Autodesk Fusion 360 part; units mm, degrees
(part 3 of 3)
  arc A621 (50.492, 81.2182) -> (50.5682, 81.142) centre (50.5682, 81.2182) ccw
  line L959 (43.8912, 86.448) -> (44.7548, 86.448)
  line L960 (109.4275, 91.606) -> (110.2911, 91.606)
  line L961 (73.826, 73.9902) -> (73.826, 74.8538)
  arc A622 (123.8293, 93.7142) -> (123.9055, 93.638) centre (123.9055, 93.7142) ccw
  line L962 (110.3673, 91.6822) -> (110.3673, 92.5458)
  arc A623 (123.9055, 96.354) -> (123.8293, 96.2778) centre (123.9055, 96.2778) ccw
  arc A624 (53.0682, 87.858) -> (52.992, 87.7818) centre (53.0682, 87.7818) ccw
  line L963 (91.401, 91.6178) -> (91.401, 90.7542)
  arc A625 (122.8133, 96.2778) -> (122.7371, 96.354) centre (122.7371, 96.2778) ccw
  arc A626 (121.8735, 94.654) -> (121.7973, 94.5778) centre (121.8735, 94.5778) ccw
  arc A627 (122.7371, 95.338) -> (122.8133, 95.4142) centre (122.7371, 95.4142) ccw
  line L964 (124.8453, 95.4142) -> (124.8453, 96.2778)
  arc A628 (52.992, 86.9182) -> (53.0682, 86.842) centre (53.0682, 86.9182) ccw
  arc A629 (122.7371, 93.638) -> (122.8133, 93.7142) centre (122.7371, 93.7142) ccw
  line L965 (123.9055, 93.638) -> (124.7691, 93.638)
  arc A630 (92.417, 91.6178) -> (92.3408, 91.694) centre (92.3408, 91.6178) ccw
  arc A631 (52.992, 85.2182) -> (53.0682, 85.142) centre (53.0682, 85.2182) ccw
  line L966 (121.8735, 93.638) -> (122.7371, 93.638)
  arc A632 (109.4275, 92.622) -> (109.3513, 92.5458) centre (109.4275, 92.5458) ccw
  line L967 (51.4318, 82.158) -> (50.5682, 82.158)
  arc A633 (91.401, 90.7542) -> (91.4772, 90.678) centre (91.4772, 90.7542) ccw
  line L968 (121.7973, 96.2778) -> (121.7973, 95.4142)
  arc A634 (89.701, 90.7542) -> (89.7772, 90.678) centre (89.7772, 90.7542) ccw
  line L969 (52.992, 87.7818) -> (52.992, 86.9182)
  arc A635 (44.7548, 86.448) -> (44.831, 86.5242) centre (44.7548, 86.5242) ccw
  line L970 (53.0682, 85.142) -> (53.9318, 85.142)
  line L971 (75.4498, 74.93) -> (74.5862, 74.93)
  line L972 (44.7548, 87.464) -> (43.8912, 87.464)
  arc A636 (43.8912, 87.464) -> (43.815, 87.3878) centre (43.8912, 87.3878) ccw
  arc A637 (75.526, 74.8538) -> (75.4498, 74.93) centre (75.4498, 74.8538) ccw
  line L973 (121.8735, 95.338) -> (122.7371, 95.338)
  arc A638 (109.4275, 94.322) -> (109.3513, 94.2458) centre (109.4275, 94.2458) ccw
  line L974 (109.3513, 94.2458) -> (109.3513, 93.3822)
  arc A639 (50.5682, 83.858) -> (50.492, 83.7818) centre (50.5682, 83.7818) ccw
  arc A640 (91.4772, 91.694) -> (91.401, 91.6178) centre (91.4772, 91.6178) ccw
  arc A641 (72.81, 73.9902) -> (72.8862, 73.914) centre (72.8862, 73.9902) ccw
  line L975 (91.4772, 90.678) -> (92.3408, 90.678)
  line L976 (109.3513, 92.5458) -> (109.3513, 91.6822)
  line L977 (124.8453, 93.7142) -> (124.8453, 94.5778)
  arc A642 (81.2292, 72.859) -> (81.153, 72.7828) centre (81.2292, 72.7828) ccw
  arc A643 (43.8912, 85.764) -> (43.815, 85.6878) centre (43.8912, 85.6878) ccw
  arc A644 (109.3513, 91.6822) -> (109.4275, 91.606) centre (109.4275, 91.6822) ccw
  line L978 (43.8912, 84.748) -> (44.7548, 84.748)
  arc A645 (110.2911, 93.306) -> (110.3673, 93.3822) centre (110.2911, 93.3822) ccw
  arc A646 (123.9055, 94.654) -> (123.8293, 94.5778) centre (123.9055, 94.5778) ccw
  line L979 (123.8293, 96.2778) -> (123.8293, 95.4142)
  line L980 (53.9318, 86.158) -> (53.0682, 86.158)
  line L981 (72.81, 74.8538) -> (72.81, 73.9902)
  arc A647 (124.8453, 96.2778) -> (124.7691, 96.354) centre (124.7691, 96.2778) ccw
  arc A648 (44.7548, 84.748) -> (44.831, 84.8242) centre (44.7548, 84.8242) ccw
  line L982 (89.7772, 90.678) -> (90.6408, 90.678)
  arc A649 (98.314, 111.517) -> (98.209, 111.412) centre (98.314, 111.412) ccw
  line L983 (120.777, 70.6492) -> (120.777, 71.5128)
  line L984 (120.7051, 94.654) -> (119.8415, 94.654)
  arc A650 (95.209, 109.822) -> (95.314, 109.717) centre (95.314, 109.822) ccw
  line L985 (120.7813, 93.7142) -> (120.7813, 94.5778)
  arc A651 (109.3513, 93.3822) -> (109.4275, 93.306) centre (109.4275, 93.3822) ccw
  line L986 (123.9055, 95.338) -> (124.7691, 95.338)
  line L987 (120.7008, 71.589) -> (119.8372, 71.589)
  arc A652 (119.8415, 94.654) -> (119.7653, 94.5778) centre (119.8415, 94.5778) ccw
  arc A653 (95.314, 111.517) -> (95.209, 111.412) centre (95.314, 111.412) ccw
  line L988 (119.761, 69.8128) -> (119.761, 68.9492)
  arc A654 (116.6009, 119.19) -> (116.7059, 119.085) centre (116.7059, 119.19) ccw
  line L989 (122.8133, 95.4142) -> (122.8133, 96.2778)
  line L990 (92.3408, 91.694) -> (91.4772, 91.694)
  arc A655 (120.7813, 94.5778) -> (120.7051, 94.654) centre (120.7051, 94.5778) ccw
  arc A656 (121.7973, 95.4142) -> (121.8735, 95.338) centre (121.8735, 95.4142) ccw
  arc A657 (119.8372, 69.889) -> (119.761, 69.8128) centre (119.8372, 69.8128) ccw
  arc A658 (120.777, 69.8128) -> (120.7008, 69.889) centre (120.7008, 69.8128) ccw
  arc A659 (119.7653, 93.7142) -> (119.8415, 93.638) centre (119.8415, 93.7142) ccw
  line L991 (90.717, 90.7542) -> (90.717, 91.6178)
  line L992 (89.701, 91.6178) -> (89.701, 90.7542)
  line L993 (122.7371, 96.354) -> (121.8735, 96.354)
  arc A660 (121.7973, 93.7142) -> (121.8735, 93.638) centre (121.8735, 93.7142) ccw
  arc A661 (124.7691, 93.638) -> (124.8453, 93.7142) centre (124.7691, 93.7142) ccw
  line L994 (98.209, 111.412) -> (98.209, 109.822)
  arc A662 (89.7772, 91.694) -> (89.701, 91.6178) centre (89.7772, 91.6178) ccw
  line L995 (124.7691, 96.354) -> (123.9055, 96.354)
  line L996 (109.4275, 93.306) -> (110.2911, 93.306)
  line L997 (119.8415, 93.638) -> (120.7051, 93.638)
  arc A663 (118.4009, 120.38) -> (118.2959, 120.485) centre (118.2959, 120.38) ccw
  line L998 (118.2959, 123.485) -> (116.7059, 123.485)
  arc A664 (116.7059, 120.485) -> (116.6009, 120.38) centre (116.7059, 120.38) ccw
  arc A665 (119.761, 68.9492) -> (119.8372, 68.873) centre (119.8372, 68.9492) ccw
  line L999 (116.7059, 122.085) -> (118.2959, 122.085)
  arc A666 (124.7691, 95.338) -> (124.8453, 95.4142) centre (124.7691, 95.4142) ccw
  arc A667 (92.3408, 90.678) -> (92.417, 90.7542) centre (92.3408, 90.7542) ccw
  line L1000 (121.7973, 94.5778) -> (121.7973, 93.7142)
  arc A668 (120.7008, 70.573) -> (120.777, 70.6492) centre (120.7008, 70.6492) ccw
  arc A669 (120.7051, 95.338) -> (120.7813, 95.4142) centre (120.7051, 95.4142) ccw
  line L1001 (122.7371, 94.654) -> (121.8735, 94.654)
  line L1002 (119.761, 71.5128) -> (119.761, 70.6492)
  arc A670 (121.8735, 96.354) -> (121.7973, 96.2778) centre (121.8735, 96.2778) ccw
  line L1003 (124.7691, 94.654) -> (123.9055, 94.654)
  arc A671 (120.777, 71.5128) -> (120.7008, 71.589) centre (120.7008, 71.5128) ccw
  line L1004 (96.504, 111.517) -> (95.314, 111.517)
  line L1005 (116.7059, 119.085) -> (118.2959, 119.085)
  arc A672 (116.7059, 123.485) -> (116.6009, 123.38) centre (116.7059, 123.38) ccw
  arc A673 (120.7051, 93.638) -> (120.7813, 93.7142) centre (120.7051, 93.7142) ccw
  line L1006 (119.8372, 70.573) -> (120.7008, 70.573)
  line L1007 (119.7653, 96.2778) -> (119.7653, 95.4142)
  line L1008 (120.777, 68.9492) -> (120.777, 69.8128)
  arc A674 (98.209, 109.822) -> (98.314, 109.717) centre (98.314, 109.822) ccw
  arc A675 (123.8293, 95.4142) -> (123.9055, 95.338) centre (123.9055, 95.4142) ccw
  arc A676 (122.8133, 94.5778) -> (122.7371, 94.654) centre (122.7371, 94.5778) ccw
  arc A677 (118.2959, 119.085) -> (118.4009, 119.19) centre (118.2959, 119.19) ccw
  arc A678 (119.8415, 96.354) -> (119.7653, 96.2778) centre (119.8415, 96.2778) ccw
  line L1009 (118.4009, 119.19) -> (118.4009, 120.38)
  line L1010 (116.6009, 123.38) -> (116.6009, 122.19)
  arc A679 (110.3673, 92.5458) -> (110.2911, 92.622) centre (110.2911, 92.5458) ccw
  line L1011 (99.609, 109.822) -> (99.609, 111.412)
  line L1012 (120.7813, 95.4142) -> (120.7813, 96.2778)
  line L1013 (122.8133, 93.7142) -> (122.8133, 94.5778)
  arc A680 (99.504, 109.717) -> (99.609, 109.822) centre (99.504, 109.822) ccw
  line L1014 (110.3673, 93.3822) -> (110.3673, 94.2458)
  line L1015 (124.7648, 69.889) -> (123.9012, 69.889)
  line L1016 (110.5408, 69.508) -> (109.6772, 69.508)
  arc A681 (116.6009, 122.19) -> (116.7059, 122.085) centre (116.7059, 122.19) ccw
  line L1017 (123.825, 71.5128) -> (123.825, 70.6492)
  line L1018 (120.7051, 96.354) -> (119.8415, 96.354)
  line L1019 (116.6009, 120.38) -> (116.6009, 119.19)
  line L1020 (79.375, 116.7502) -> (79.375, 117.6138)
  arc A682 (79.375, 117.6138) -> (79.2988, 117.69) centre (79.2988, 117.6138) ccw
  arc A683 (78.4352, 117.69) -> (78.359, 117.6138) centre (78.4352, 117.6138) ccw
  line L1021 (120.7008, 69.889) -> (119.8372, 69.889)
  line L1022 (109.6772, 68.492) -> (110.5408, 68.492)
  arc A684 (123.825, 70.6492) -> (123.9012, 70.573) centre (123.9012, 70.6492) ccw
  line L1023 (95.209, 111.412) -> (95.209, 109.822)
  arc A685 (120.7008, 68.873) -> (120.777, 68.9492) centre (120.7008, 68.9492) ccw
  arc A686 (96.609, 111.412) -> (96.504, 111.517) centre (96.504, 111.412) ccw
  line L1024 (118.2959, 120.485) -> (116.7059, 120.485)
  arc A687 (78.359, 116.7502) -> (78.4352, 116.674) centre (78.4352, 116.7502) ccw
  arc A688 (124.841, 69.8128) -> (124.7648, 69.889) centre (124.7648, 69.8128) ccw
  line L1025 (121.8692, 70.573) -> (122.7328, 70.573)
  line L1026 (96.609, 109.822) -> (96.609, 111.412)
  arc A689 (110.2911, 91.606) -> (110.3673, 91.6822) centre (110.2911, 91.6822) ccw
  arc A690 (121.8692, 69.889) -> (121.793, 69.8128) centre (121.8692, 69.8128) ccw
  line L1027 (124.841, 70.6492) -> (124.841, 71.5128)
  arc A691 (121.8692, 71.589) -> (121.793, 71.5128) centre (121.8692, 71.5128) ccw
  arc A692 (109.6772, 69.508) -> (109.601, 69.4318) centre (109.6772, 69.4318) ccw
  arc A693 (124.7648, 70.573) -> (124.841, 70.6492) centre (124.7648, 70.6492) ccw
  arc A694 (110.5408, 68.492) -> (110.617, 68.5682) centre (110.5408, 68.5682) ccw
  arc A695 (96.504, 109.717) -> (96.609, 109.822) centre (96.504, 109.822) ccw
  line L1028 (124.7648, 71.589) -> (123.9012, 71.589)
  line L1029 (122.7328, 69.889) -> (121.8692, 69.889)
  line L1030 (119.8415, 95.338) -> (120.7051, 95.338)
  line L1031 (110.617, 68.5682) -> (110.617, 69.4318)
  line L1032 (118.4009, 122.19) -> (118.4009, 123.38)
  line L1033 (121.793, 71.5128) -> (121.793, 70.6492)
  line L1034 (99.504, 111.517) -> (98.314, 111.517)
  arc A696 (119.761, 70.6492) -> (119.8372, 70.573) centre (119.8372, 70.6492) ccw
  arc A697 (122.7328, 68.873) -> (122.809, 68.9492) centre (122.7328, 68.9492) ccw
  arc A698 (99.609, 111.412) -> (99.504, 111.517) centre (99.504, 111.412) ccw
  line L1035 (119.7653, 94.5778) -> (119.7653, 93.7142)
  arc A699 (119.7653, 95.4142) -> (119.8415, 95.338) centre (119.8415, 95.4142) ccw
  arc A700 (123.825, 68.9492) -> (123.9012, 68.873) centre (123.9012, 68.9492) ccw
  line L1036 (78.359, 115.9138) -> (78.359, 115.0502)
  line L1037 (109.6772, 70.192) -> (110.5408, 70.192)
  arc A701 (119.8372, 71.589) -> (119.761, 71.5128) centre (119.8372, 71.5128) ccw
  arc A702 (118.2959, 122.085) -> (118.4009, 122.19) centre (118.2959, 122.19) ccw
  arc A703 (123.9012, 71.589) -> (123.825, 71.5128) centre (123.9012, 71.5128) ccw
  arc A704 (109.601, 68.5682) -> (109.6772, 68.492) centre (109.6772, 68.5682) ccw
  line L1038 (98.314, 109.717) -> (99.504, 109.717)
  arc A705 (121.793, 68.9492) -> (121.8692, 68.873) centre (121.8692, 68.9492) ccw
  arc A706 (109.6772, 71.208) -> (109.601, 71.1318) centre (109.6772, 71.1318) ccw
  line L1039 (95.314, 109.717) -> (96.504, 109.717)
  line L1040 (78.4352, 114.974) -> (79.2988, 114.974)
  arc A707 (118.4009, 123.38) -> (118.2959, 123.485) centre (118.2959, 123.38) ccw
  arc A708 (78.4352, 115.99) -> (78.359, 115.9138) centre (78.4352, 115.9138) ccw
  arc A709 (78.359, 115.0502) -> (78.4352, 114.974) centre (78.4352, 115.0502) ccw
  line L1041 (123.9012, 68.873) -> (124.7648, 68.873)
  line L1042 (122.809, 68.9492) -> (122.809, 69.8128)
  line L1043 (122.7328, 71.589) -> (121.8692, 71.589)
  line L1044 (109.601, 71.1318) -> (109.601, 70.2682)
  arc A710 (124.841, 71.5128) -> (124.7648, 71.589) centre (124.7648, 71.5128) ccw
  line L1045 (119.8372, 68.873) -> (120.7008, 68.873)
  arc A711 (120.7813, 96.2778) -> (120.7051, 96.354) centre (120.7051, 96.2778) ccw
  line L1046 (121.793, 69.8128) -> (121.793, 68.9492)
  line L1047 (79.2988, 117.69) -> (78.4352, 117.69)
  line L1048 (66.928, 77.135) -> (66.028, 77.135)
  line L1049 (46.909, 73.405) -> (46.309, 73.405)
  line L1050 (47.859, 71.005) -> (47.259, 71.005)
  line L1051 (63.628, 78.085) -> (63.628, 77.485)
  arc A712 (110.5408, 70.192) -> (110.617, 70.2682) centre (110.5408, 70.2682) ccw
  line L1052 (45.959, 71.005) -> (45.359, 71.005)
  line L1053 (83.914, 118.45) -> (85.504, 118.45)
  line L1054 (46.309, 72.505) -> (46.909, 72.505)
  line L1055 (45.359, 70.105) -> (45.959, 70.105)
  arc A713 (85.504, 121.45) -> (85.609, 121.555) centre (85.504, 121.555) ccw
  line L1056 (46.25, 81.25) -> (45.65, 81.25)
  line L1057 (109.601, 69.4318) -> (109.601, 68.5682)
  arc A714 (121.793, 70.6492) -> (121.8692, 70.573) centre (121.8692, 70.6492) ccw
  arc A715 (110.617, 71.1318) -> (110.5408, 71.208) centre (110.5408, 71.1318) ccw
  arc A716 (122.809, 71.5128) -> (122.7328, 71.589) centre (122.7328, 71.5128) ccw
  line L1058 (78.4352, 116.674) -> (79.2988, 116.674)
  line L1059 (66.028, 76.185) -> (66.028, 75.585)
  line L1060 (110.617, 70.2682) -> (110.617, 71.1318)
  line L1061 (66.028, 76.535) -> (66.928, 76.535)
  arc A717 (66.628, 77.485) -> (66.628, 78.085) centre (66.628, 77.785) ccw
  line L1062 (66.028, 77.135) -> (66.028, 76.535)
  line L1063 (122.809, 70.6492) -> (122.809, 71.5128)
  line L1064 (63.628, 77.485) -> (64.528, 77.485)
  line L1065 (46.909, 72.505) -> (46.909, 73.405)
  arc A718 (109.601, 70.2682) -> (109.6772, 70.192) centre (109.6772, 70.2682) ccw
  line L1066 (123.9012, 70.573) -> (124.7648, 70.573)
  line L1067 (47.259, 73.405) -> (47.259, 72.505)
  line L1068 (43.75, 80.35) -> (44.35, 80.35)
  line L1069 (124.841, 68.9492) -> (124.841, 69.8128)
  line L1070 (123.825, 69.8128) -> (123.825, 68.9492)
  line L1071 (121.8692, 68.873) -> (122.7328, 68.873)
  arc A719 (122.809, 69.8128) -> (122.7328, 69.889) centre (122.7328, 69.8128) ccw
  line L1072 (63.628, 75.585) -> (64.528, 75.585)
  arc A720 (124.7648, 68.873) -> (124.841, 68.9492) centre (124.7648, 68.9492) ccw
  arc A721 (83.809, 118.555) -> (83.914, 118.45) centre (83.914, 118.555) ccw
  line L1073 (45.359, 72.805) -> (45.359, 73.105)
  line L1074 (64.528, 78.085) -> (63.628, 78.085)
  arc A722 (123.9012, 69.889) -> (123.825, 69.8128) centre (123.9012, 69.8128) ccw
  arc A723 (110.617, 69.4318) -> (110.5408, 69.508) centre (110.5408, 69.4318) ccw
  line L1075 (47.859, 73.405) -> (47.259, 73.405)
  line L1076 (110.5408, 71.208) -> (109.6772, 71.208)
  arc A724 (83.809, 121.555) -> (83.914, 121.45) centre (83.914, 121.555) ccw
  arc A725 (122.7328, 70.573) -> (122.809, 70.6492) centre (122.7328, 70.6492) ccw
  arc A726 (85.609, 119.745) -> (85.504, 119.85) centre (85.504, 119.745) ccw
  line L1077 (79.2988, 115.99) -> (78.4352, 115.99)
  line L1078 (78.359, 117.6138) -> (78.359, 116.7502)
  line L1079 (45.959, 72.805) -> (45.959, 73.105)
  line L1080 (64.528, 75.585) -> (64.528, 76.185)
  line L1081 (85.609, 121.555) -> (85.609, 122.745)
  line L1082 (47.859, 70.105) -> (47.859, 71.005)
  line L1083 (66.328, 78.085) -> (66.628, 78.085)
  line L1084 (66.328, 77.485) -> (66.628, 77.485)
  line L1085 (79.375, 115.0502) -> (79.375, 115.9138)
  line L1086 (83.809, 122.745) -> (83.809, 121.555)
  line L1087 (66.028, 75.585) -> (66.928, 75.585)
  line L1088 (64.528, 77.485) -> (64.528, 78.085)
  line L1089 (47.259, 70.105) -> (47.859, 70.105)
  line L1090 (66.928, 76.535) -> (66.928, 77.135)
  arc A727 (79.2988, 116.674) -> (79.375, 116.7502) centre (79.2988, 116.7502) ccw
  arc A728 (45.959, 73.105) -> (45.359, 73.105) centre (45.659, 73.105) ccw
  line L1091 (85.504, 119.85) -> (83.914, 119.85)
  line L1092 (64.528, 76.185) -> (63.628, 76.185)
  line L1093 (46.309, 73.405) -> (46.309, 72.505)
  line L1094 (63.628, 76.185) -> (63.628, 75.585)
  line L1095 (119.4533, 90.99) -> (119.8533, 90.59)
  line L1096 (73.337, 51.5835) -> (73.337, 51.1585)
  arc A729 (85.609, 122.745) -> (85.504, 122.85) centre (85.504, 122.745) ccw
  line L1097 (74.237, 51.5835) -> (74.0245, 51.796)
  arc A730 (44.35, 83.35) -> (43.75, 83.35) centre (44.05, 83.35) ccw
  line L1098 (47.859, 72.505) -> (47.859, 73.405)
  line L1099 (74.0245, 50.946) -> (74.237, 51.1585)
  line L1100 (44.7, 83.65) -> (44.7, 82.75)
  line L1101 (46.25, 82.75) -> (46.25, 83.65)
  line L1102 (46.25, 80.35) -> (46.25, 81.25)
  line L1103 (83.775, 87.675) -> (84.225, 87.675)
  line L1104 (75.623, 50.146) -> (75.623, 49.296)
  line L1105 (75.623, 51.5835) -> (75.623, 51.1585)
  line L1106 (85.504, 122.85) -> (83.914, 122.85)
  line L1107 (73.337, 50.146) -> (73.337, 49.296)
  arc A731 (45.359, 72.805) -> (45.959, 72.805) centre (45.659, 72.805) ccw
  line L1108 (124.9033, 90.59) -> (124.9033, 92.29)
  line L1109 (84.225, 87.675) -> (84.45, 87.9)
  line L1110 (83.775, 88.575) -> (83.55, 88.35)
  line L1111 (84.45, 85.325) -> (83.55, 85.325)
  line L1112 (45.959, 70.105) -> (45.959, 71.005)
  line L1113 (84.45, 84.425) -> (84.45, 85.325)
  line L1114 (43.75, 83.05) -> (43.75, 83.35)
  line L1115 (45.3, 83.65) -> (44.7, 83.65)
  arc A732 (83.914, 119.85) -> (83.809, 119.745) centre (83.914, 119.745) ccw
  line L1116 (74.237, 51.1585) -> (74.237, 51.5835)
  line L1117 (75.8355, 51.796) -> (75.623, 51.5835)
  line L1118 (76.523, 51.1585) -> (76.523, 51.5835)
  line L1119 (83.55, 87.9) -> (83.775, 87.675)
  line L1120 (45.65, 80.35) -> (46.25, 80.35)
  line L1121 (83.55, 85.325) -> (83.55, 84.425)
  line L1122 (45.65, 83.65) -> (45.65, 82.75)
  arc A733 (83.914, 122.85) -> (83.809, 122.745) centre (83.914, 122.745) ccw
  line L1123 (43.75, 81.25) -> (43.75, 80.35)
  line L1124 (45.65, 82.75) -> (46.25, 82.75)
  arc A734 (79.375, 115.9138) -> (79.2988, 115.99) centre (79.2988, 115.9138) ccw
  line L1125 (45.65, 81.25) -> (45.65, 80.35)
  line L1126 (73.5495, 51.796) -> (73.337, 51.5835)
  line L1127 (76.523, 51.5835) -> (76.3105, 51.796)
  line L1128 (44.35, 81.25) -> (43.75, 81.25)
  line L1129 (85.609, 118.555) -> (85.609, 119.745)
  arc A735 (79.2988, 114.974) -> (79.375, 115.0502) centre (79.2988, 115.0502) ccw
  line L1130 (76.3105, 51.796) -> (75.8355, 51.796)
  line L1131 (83.55, 84.425) -> (84.45, 84.425)
  line L1132 (74.237, 49.296) -> (74.237, 50.146)
  line L1133 (75.8355, 50.946) -> (76.3105, 50.946)
  line L1134 (83.55, 88.35) -> (83.55, 87.9)
  line L1135 (47.259, 71.005) -> (47.259, 70.105)
  line L1136 (44.35, 80.35) -> (44.35, 81.25)
  line L1137 (44.7, 82.75) -> (45.3, 82.75)
  line L1138 (120.6533, 90.59) -> (121.0533, 90.99)
  line L1139 (45.3, 82.75) -> (45.3, 83.65)
  line L1140 (66.928, 76.185) -> (66.028, 76.185)
  line L1141 (45.359, 71.005) -> (45.359, 70.105)
  line L1142 (76.523, 49.296) -> (76.523, 50.146)
  arc A736 (66.328, 78.085) -> (66.328, 77.485) centre (66.328, 77.785) ccw
  line L1143 (84.45, 87.9) -> (84.45, 88.35)
  line L1144 (66.928, 75.585) -> (66.928, 76.185)
  line L1145 (83.809, 119.745) -> (83.809, 118.555)
  line L1146 (47.259, 72.505) -> (47.859, 72.505)
  line L1147 (83.914, 121.45) -> (85.504, 121.45)
  arc A737 (85.504, 118.45) -> (85.609, 118.555) centre (85.504, 118.555) ccw
  line L1148 (46.25, 83.65) -> (45.65, 83.65)
  line L1149 (76.3105, 50.946) -> (76.523, 51.1585)
  arc A738 (47.2313, 67.5443) -> (47.3513, 67.4243) centre (47.3513, 67.5443) ccw
  line L1150 (60.815, 120.2) -> (61.215, 119.8)
  line L1151 (61.215, 119.8) -> (62.015, 119.8)
  line L1152 (68.111, 76.2508) -> (68.111, 75.3872)
  line L1153 (121.049, 66.225) -> (121.049, 67.125)
  line L1154 (75.623, 51.1585) -> (75.8355, 50.946)
  line L1155 (119.8533, 90.59) -> (120.6533, 90.59)
  line L1156 (123.3033, 92.29) -> (123.3033, 90.59)
  arc A739 (44.3865, 67.5443) -> (44.5065, 67.4243) centre (44.5065, 67.5443) ccw
  line L1157 (119.4533, 91.89) -> (119.4533, 90.99)
  line L1158 (87.968, 70.935) -> (87.968, 70.035)
  line L1159 (73.5495, 50.946) -> (74.0245, 50.946)
  line L1160 (73.337, 49.296) -> (74.237, 49.296)
  line L1161 (62.415, 120.2) -> (62.415, 121.1)
  line L1162 (124.899, 65.825) -> (124.899, 67.525)
  arc A740 (43.75, 83.05) -> (44.35, 83.05) centre (44.05, 83.05) ccw
  line L1163 (91.893, 70.035) -> (92.118, 70.26)
  line L1164 (91.893, 70.935) -> (91.443, 70.935)
  line L1165 (47.3513, 67.4243) -> (48.7115, 67.4243)
  arc A741 (48.8315, 69.1077) -> (48.7115, 69.2277) centre (48.7115, 69.1077) ccw
  line L1166 (124.9033, 92.29) -> (123.3033, 92.29)
  line L1167 (44.5065, 67.4243) -> (45.8667, 67.4243)
  arc A742 (69.8872, 76.327) -> (69.811, 76.2508) centre (69.8872, 76.2508) ccw
  line L1168 (92.118, 70.71) -> (91.893, 70.935)
  line L1169 (47.2313, 69.1077) -> (47.2313, 67.5443)
  line L1170 (121.0533, 90.99) -> (121.0533, 91.89)
  line L1171 (76.523, 50.146) -> (75.623, 50.146)
  line L1172 (58.565, 121.5) -> (56.965, 121.5)
  line L1173 (123.299, 67.525) -> (123.299, 65.825)
  arc A743 (70.7508, 75.311) -> (70.827, 75.3872) centre (70.7508, 75.3872) ccw
  line L1174 (121.0533, 91.89) -> (120.6533, 92.29)
  arc A744 (69.811, 75.3872) -> (69.8872, 75.311) centre (69.8872, 75.3872) ccw
  line L1175 (48.7115, 69.2277) -> (47.3513, 69.2277)
  arc A745 (70.827, 76.2508) -> (70.7508, 76.327) centre (70.7508, 76.2508) ccw
  line L1176 (74.237, 50.146) -> (73.337, 50.146)
  line L1177 (74.0245, 51.796) -> (73.5495, 51.796)
  line L1178 (119.449, 66.225) -> (119.849, 65.825)
  line L1179 (48.8315, 67.5443) -> (48.8315, 69.1077)
  line L1180 (68.1872, 75.311) -> (69.0508, 75.311)
  line L1181 (119.849, 67.525) -> (119.449, 67.125)
  line L1182 (88.868, 70.035) -> (88.868, 70.935)
  line L1183 (70.827, 75.3872) -> (70.827, 76.2508)
  line L1184 (120.649, 67.525) -> (119.849, 67.525)
  line L1185 (124.899, 67.525) -> (123.299, 67.525)
  arc A746 (47.3513, 69.2277) -> (47.2313, 69.1077) centre (47.3513, 69.1077) ccw
  line L1186 (120.6533, 92.29) -> (119.8533, 92.29)
  line L1187 (44.35, 83.05) -> (44.35, 83.35)
  line L1188 (60.815, 121.1) -> (60.815, 120.2)
  line L1189 (62.415, 121.1) -> (62.015, 121.5)
  line L1190 (84.45, 88.35) -> (84.225, 88.575)
  line L1191 (73.337, 51.1585) -> (73.5495, 50.946)
  line L1192 (88.868, 70.935) -> (87.968, 70.935)
  line L1193 (84.225, 88.575) -> (83.775, 88.575)
  arc A747 (45.9867, 69.1077) -> (45.8667, 69.2277) centre (45.8667, 69.1077) ccw
  line L1194 (92.118, 70.26) -> (92.118, 70.71)
  line L1195 (87.968, 70.035) -> (88.868, 70.035)
  line L1196 (62.015, 119.8) -> (62.415, 120.2)
  line L1197 (75.623, 49.296) -> (76.523, 49.296)
  arc A748 (48.7115, 67.4243) -> (48.8315, 67.5443) centre (48.7115, 67.5443) ccw
  line L1198 (91.218, 70.26) -> (91.443, 70.035)
  line L1199 (119.8533, 92.29) -> (119.4533, 91.89)
  line L1200 (69.127, 75.3872) -> (69.127, 76.2508)
  line L1201 (123.3033, 90.59) -> (124.9033, 90.59)
  line L1202 (69.0508, 76.327) -> (68.1872, 76.327)
  arc A749 (44.8777, 79.2817) -> (44.7577, 79.4017) centre (44.7577, 79.2817) ccw
  arc A750 (72.556, 68.0838) -> (72.4798, 68.16) centre (72.4798, 68.0838) ccw
  line L1203 (58.565, 119.8) -> (58.565, 121.5)
  line L1204 (43.2775, 79.2817) -> (43.2775, 77.7183)
  arc A751 (83.0598, 65.024) -> (83.136, 65.1002) centre (83.0598, 65.1002) ccw
  line L1205 (69.8872, 75.311) -> (70.7508, 75.311)
  line L1206 (45.9867, 67.5443) -> (45.9867, 69.1077)
  arc A752 (83.8962, 66.04) -> (83.82, 65.9638) centre (83.8962, 65.9638) ccw
  line L1207 (123.299, 65.825) -> (124.899, 65.825)
  arc A753 (71.6162, 66.46) -> (71.54, 66.3838) centre (71.6162, 66.3838) ccw
  arc A754 (47.7225, 79.2817) -> (47.6025, 79.4017) centre (47.6025, 79.2817) ccw
  arc A755 (82.12, 65.1002) -> (82.1962, 65.024) centre (82.1962, 65.1002) ccw
  line L1208 (83.8962, 67.564) -> (84.7598, 67.564)
  arc A756 (84.7598, 65.024) -> (84.836, 65.1002) centre (84.7598, 65.1002) ccw
  line L1209 (72.556, 67.2202) -> (72.556, 68.0838)
  arc A757 (82.1962, 68.58) -> (82.12, 68.5038) centre (82.1962, 68.5038) ccw
  line L1210 (84.836, 65.1002) -> (84.836, 65.9638)
  line L1211 (43.3975, 77.5983) -> (44.7577, 77.5983)
  line L1212 (121.049, 67.125) -> (120.649, 67.525)
  arc A758 (69.127, 76.2508) -> (69.0508, 76.327) centre (69.0508, 76.2508) ccw
  line L1213 (70.7508, 76.327) -> (69.8872, 76.327)
  arc A759 (82.12, 67.6402) -> (82.1962, 67.564) centre (82.1962, 67.6402) ccw
  line L1214 (119.849, 65.825) -> (120.649, 65.825)
  arc A760 (71.54, 65.5202) -> (71.6162, 65.444) centre (71.6162, 65.5202) ccw
  arc A761 (45.8667, 67.4243) -> (45.9867, 67.5443) centre (45.8667, 67.5443) ccw
  line L1215 (82.1962, 67.564) -> (83.0598, 67.564)
  line L1216 (83.82, 65.9638) -> (83.82, 65.1002)
  line L1217 (91.218, 70.71) -> (91.218, 70.26)
  line L1218 (71.6162, 65.444) -> (72.4798, 65.444)
  line L1219 (69.811, 76.2508) -> (69.811, 75.3872)
  arc A762 (43.2775, 77.7183) -> (43.3975, 77.5983) centre (43.3975, 77.7183) ccw
  arc A763 (68.111, 75.3872) -> (68.1872, 75.311) centre (68.1872, 75.3872) ccw
  line L1220 (91.443, 70.935) -> (91.218, 70.71)
  line L1221 (82.12, 68.5038) -> (82.12, 67.6402)
  line L1222 (72.556, 65.5202) -> (72.556, 66.3838)
  line L1223 (56.965, 119.8) -> (58.565, 119.8)
  line L1224 (83.82, 68.5038) -> (83.82, 67.6402)
  line L1225 (62.015, 121.5) -> (61.215, 121.5)
  line L1226 (72.4798, 68.16) -> (71.6162, 68.16)
  arc A764 (83.136, 65.9638) -> (83.0598, 66.04) centre (83.0598, 65.9638) ccw
  arc A765 (83.136, 68.5038) -> (83.0598, 68.58) centre (83.0598, 68.5038) ccw
  line L1227 (45.8667, 69.2277) -> (44.5065, 69.2277)
  line L1228 (84.7598, 68.58) -> (83.8962, 68.58)
  arc A766 (46.1223, 77.7183) -> (46.2423, 77.5983) centre (46.2423, 77.7183) ccw
  line L1229 (83.0598, 68.58) -> (82.1962, 68.58)
  arc A767 (69.0508, 75.311) -> (69.127, 75.3872) centre (69.0508, 75.3872) ccw
  arc A768 (47.6025, 77.5983) -> (47.7225, 77.7183) centre (47.6025, 77.7183) ccw
  line L1230 (91.443, 70.035) -> (91.893, 70.035)
  line L1231 (46.1223, 79.2817) -> (46.1223, 77.7183)
  arc A769 (46.2423, 79.4017) -> (46.1223, 79.2817) centre (46.2423, 79.2817) ccw
  arc A770 (72.4798, 67.144) -> (72.556, 67.2202) centre (72.4798, 67.2202) ccw
  arc A771 (71.6162, 68.16) -> (71.54, 68.0838) centre (71.6162, 68.0838) ccw
  line L1232 (83.136, 67.6402) -> (83.136, 68.5038)
  line L1233 (71.54, 66.3838) -> (71.54, 65.5202)
  arc A772 (83.0598, 67.564) -> (83.136, 67.6402) centre (83.0598, 67.6402) ccw
  line L1234 (84.836, 67.6402) -> (84.836, 68.5038)
  line L1235 (83.136, 65.1002) -> (83.136, 65.9638)
  line L1236 (44.3865, 69.1077) -> (44.3865, 67.5443)
  arc A773 (44.5065, 69.2277) -> (44.3865, 69.1077) centre (44.5065, 69.1077) ccw
  line L1237 (56.965, 121.5) -> (56.965, 119.8)
  line L1238 (119.449, 67.125) -> (119.449, 66.225)
  line L1239 (120.649, 65.825) -> (121.049, 66.225)
  line L1240 (61.215, 121.5) -> (60.815, 121.1)
  arc A774 (43.3975, 79.4017) -> (43.2775, 79.2817) centre (43.3975, 79.2817) ccw
  arc A775 (114.173, 97.5732) -> (114.2492, 97.497) centre (114.2492, 97.5732) ccw
  line L1241 (113.2967, 95.6875) -> (113.2967, 97.0477)
  line L1242 (82.12, 65.9638) -> (82.12, 65.1002)
  arc A776 (111.6133, 97.1677) -> (111.4933, 97.0477) centre (111.6133, 97.0477) ccw
  line L1243 (93.2223, 93.3568) -> (93.2223, 92.4932)
  line L1244 (83.0598, 66.04) -> (82.1962, 66.04)
  line L1245 (114.173, 98.4368) -> (114.173, 97.5732)
  line L1246 (107.7595, 119.7807) -> (107.7595, 118.2173)
  arc A777 (83.8962, 68.58) -> (83.82, 68.5038) centre (83.8962, 68.5038) ccw
  line L1247 (83.8962, 65.024) -> (84.7598, 65.024)
  line L1248 (109.3597, 118.2173) -> (109.3597, 119.7807)
  line L1249 (115.1128, 98.513) -> (114.2492, 98.513)
  arc A778 (94.2383, 93.3568) -> (94.1621, 93.433) centre (94.1621, 93.3568) ccw
  line L1250 (44.7577, 79.4017) -> (43.3975, 79.4017)
  line L1251 (94.2383, 92.4932) -> (94.2383, 93.3568)
  arc A779 (83.82, 65.1002) -> (83.8962, 65.024) centre (83.8962, 65.1002) ccw
  arc A780 (113.1767, 98.4123) -> (113.2967, 98.5323) centre (113.1767, 98.5323) ccw
  arc A781 (115.1128, 95.797) -> (115.189, 95.8732) centre (115.1128, 95.8732) ccw
  arc A782 (115.189, 96.7368) -> (115.1128, 96.813) centre (115.1128, 96.7368) ccw
  arc A783 (114.173, 95.8732) -> (114.2492, 95.797) centre (114.2492, 95.8732) ccw
  arc A784 (84.836, 65.9638) -> (84.7598, 66.04) centre (84.7598, 65.9638) ccw
  arc A785 (94.1621, 92.417) -> (94.2383, 92.4932) centre (94.1621, 92.4932) ccw
  line L1252 (115.189, 95.8732) -> (115.189, 96.7368)
  arc A786 (83.82, 67.6402) -> (83.8962, 67.564) centre (83.8962, 67.6402) ccw
  arc A787 (68.1872, 76.327) -> (68.111, 76.2508) centre (68.1872, 76.2508) ccw
  line L1253 (93.2985, 90.717) -> (94.1621, 90.717)
  arc A788 (114.2492, 96.813) -> (114.173, 96.7368) centre (114.2492, 96.7368) ccw
  line L1254 (94.1621, 93.433) -> (93.2985, 93.433)
  line L1255 (107.8795, 118.0973) -> (109.2397, 118.0973)
  line L1256 (113.2967, 98.5323) -> (113.2967, 99.8925)
  line L1257 (110.7243, 118.0973) -> (112.0845, 118.0973)
  arc A789 (84.836, 68.5038) -> (84.7598, 68.58) centre (84.7598, 68.5038) ccw
  arc A790 (71.54, 67.2202) -> (71.6162, 67.144) centre (71.6162, 67.2202) ccw
  line L1258 (71.6162, 67.144) -> (72.4798, 67.144)
  arc A791 (93.2985, 91.733) -> (93.2223, 91.6568) centre (93.2985, 91.6568) ccw
  arc A792 (44.7577, 77.5983) -> (44.8777, 77.7183) centre (44.7577, 77.7183) ccw
  arc A793 (107.8795, 119.9007) -> (107.7595, 119.7807) centre (107.8795, 119.7807) ccw
  line L1259 (93.2223, 91.6568) -> (93.2223, 90.7932)
  line L1260 (111.6133, 95.5675) -> (113.1767, 95.5675)
  line L1261 (46.2423, 77.5983) -> (47.6025, 77.5983)
  line L1262 (110.6043, 119.7807) -> (110.6043, 118.2173)
  line L1263 (84.7598, 66.04) -> (83.8962, 66.04)
  arc A794 (93.2223, 92.4932) -> (93.2985, 92.417) centre (93.2985, 92.4932) ccw
  line L1264 (112.0845, 119.9007) -> (110.7243, 119.9007)
  arc A795 (109.2397, 118.0973) -> (109.3597, 118.2173) centre (109.2397, 118.2173) ccw
  arc A796 (111.4933, 98.5323) -> (111.6133, 98.4123) centre (111.6133, 98.5323) ccw
  line L1265 (115.1128, 96.813) -> (114.2492, 96.813)
  line L1266 (47.7225, 77.7183) -> (47.7225, 79.2817)
  line L1267 (82.1962, 65.024) -> (83.0598, 65.024)
  line L1268 (111.6133, 98.4123) -> (113.1767, 98.4123)
  arc A797 (113.2967, 99.8925) -> (113.1767, 100.0125) centre (113.1767, 99.8925) ccw
  arc A798 (94.1621, 90.717) -> (94.2383, 90.7932) centre (94.1621, 90.7932) ccw
  line L1269 (44.8777, 77.7183) -> (44.8777, 79.2817)
  arc A799 (82.1962, 66.04) -> (82.12, 65.9638) centre (82.1962, 65.9638) ccw
  arc A800 (107.7595, 118.2173) -> (107.8795, 118.0973) centre (107.8795, 118.2173) ccw
  arc A801 (109.3597, 119.7807) -> (109.2397, 119.9007) centre (109.2397, 119.7807) ccw
  line L1270 (112.2045, 118.2173) -> (112.2045, 119.7807)
  line L1271 (47.6025, 79.4017) -> (46.2423, 79.4017)
  arc A802 (72.4798, 65.444) -> (72.556, 65.5202) centre (72.4798, 65.5202) ccw
  line L1272 (72.4798, 66.46) -> (71.6162, 66.46)
  arc A803 (72.556, 66.3838) -> (72.4798, 66.46) centre (72.4798, 66.3838) ccw
  line L1273 (71.54, 68.0838) -> (71.54, 67.2202)
  arc A804 (93.2985, 93.433) -> (93.2223, 93.3568) centre (93.2985, 93.3568) ccw
  line L1274 (109.2397, 119.9007) -> (107.8795, 119.9007)
  line L1275 (113.1767, 73.7997) -> (111.6133, 73.7997)
  arc A805 (115.1128, 72.429) -> (115.189, 72.5052) centre (115.1128, 72.5052) ccw
  arc A806 (111.4933, 95.6875) -> (111.6133, 95.5675) centre (111.6133, 95.6875) ccw
  arc A807 (113.2967, 97.0477) -> (113.1767, 97.1677) centre (113.1767, 97.0477) ccw
  line L1276 (116.7695, 113.3478) -> (118.1297, 113.3478)
  line L1277 (111.4933, 76.5245) -> (111.4933, 75.1643)
  arc A808 (114.173, 72.5052) -> (114.2492, 72.429) centre (114.2492, 72.5052) ccw
  line L1278 (94.1621, 91.733) -> (93.2985, 91.733)
  arc A809 (94.615, 70.0142) -> (94.6912, 69.938) centre (94.6912, 70.0142) ccw
  line L1279 (94.615, 69.1778) -> (94.615, 68.3142)
  line L1280 (93.2985, 92.417) -> (94.1621, 92.417)
  line L1281 (116.6495, 115.0311) -> (116.6495, 113.4678)
  line L1282 (94.2383, 90.7932) -> (94.2383, 91.6568)
  line L1283 (94.6912, 68.238) -> (95.5548, 68.238)
  arc A810 (121.0945, 115.0311) -> (120.9745, 115.1512) centre (120.9745, 115.0311) ccw
  line L1284 (113.2967, 75.1643) -> (113.2967, 76.5245)
  line L1285 (118.1297, 115.1512) -> (116.7695, 115.1512)
  arc A811 (114.2492, 73.445) -> (114.173, 73.3688) centre (114.2492, 73.3688) ccw
  arc A812 (95.631, 70.8778) -> (95.5548, 70.954) centre (95.5548, 70.8778) ccw
  line L1286 (95.631, 70.0142) -> (95.631, 70.8778)
  arc A813 (111.6133, 73.7997) -> (111.4933, 73.6797) centre (111.6133, 73.6797) ccw
  arc A814 (111.4933, 72.3195) -> (111.6133, 72.1995) centre (111.6133, 72.3195) ccw
  line L1287 (95.631, 68.3142) -> (95.631, 69.1778)
  line L1288 (111.6133, 75.0443) -> (113.1767, 75.0443)
  arc A815 (115.1128, 74.129) -> (115.189, 74.2052) centre (115.1128, 74.2052) ccw
  line L1289 (94.6912, 69.938) -> (95.5548, 69.938)
  arc A816 (111.6133, 100.0125) -> (111.4933, 99.8925) centre (111.6133, 99.8925) ccw
  line L1290 (115.189, 97.5732) -> (115.189, 98.4368)
  line L1291 (94.615, 70.8778) -> (94.615, 70.0142)
  line L1292 (113.1767, 100.0125) -> (111.6133, 100.0125)
  arc A817 (113.1767, 75.0443) -> (113.2967, 75.1643) centre (113.1767, 75.1643) ccw
  arc A818 (114.2492, 98.513) -> (114.173, 98.4368) centre (114.2492, 98.4368) ccw
  arc A819 (113.1767, 95.5675) -> (113.2967, 95.6875) centre (113.1767, 95.6875) ccw
  arc A820 (115.1128, 97.497) -> (115.189, 97.5732) centre (115.1128, 97.5732) ccw
  line L1293 (111.4933, 99.8925) -> (111.4933, 98.5323)
  line L1294 (114.2492, 72.429) -> (115.1128, 72.429)
  line L1295 (95.5548, 69.254) -> (94.6912, 69.254)
  line L1296 (114.2492, 97.497) -> (115.1128, 97.497)
  line L1297 (118.2497, 113.4678) -> (118.2497, 115.0311)
  line L1298 (114.173, 96.7368) -> (114.173, 95.8732)
  arc A821 (95.5548, 69.938) -> (95.631, 70.0142) centre (95.5548, 70.0142) ccw
  arc A822 (111.6133, 76.6445) -> (111.4933, 76.5245) centre (111.6133, 76.5245) ccw
  line L1299 (113.1767, 97.1677) -> (111.6133, 97.1677)
  line L1300 (114.2492, 95.797) -> (115.1128, 95.797)
  arc A823 (93.2223, 90.7932) -> (93.2985, 90.717) centre (93.2985, 90.7932) ccw
  arc A824 (118.1297, 113.3478) -> (118.2497, 113.4678) centre (118.1297, 113.4678) ccw
  arc A825 (115.189, 98.4368) -> (115.1128, 98.513) centre (115.1128, 98.4368) ccw
  arc A826 (84.7598, 67.564) -> (84.836, 67.6402) centre (84.7598, 67.6402) ccw
  arc A827 (110.6043, 118.2173) -> (110.7243, 118.0973) centre (110.7243, 118.2173) ccw
  arc A828 (94.2383, 91.6568) -> (94.1621, 91.733) centre (94.1621, 91.6568) ccw
  line L1301 (111.4933, 97.0477) -> (111.4933, 95.6875)
  arc A829 (119.6143, 115.1512) -> (119.4943, 115.0311) centre (119.6143, 115.0311) ccw
  line L1302 (30, 131) -> (190.5, 131)
  line L1303 (190.5, 131) -> (190.5, 41.6961)
  line L1304 (190.5, 41.6961) -> (30, 41.6961)
  line L1305 (30, 41.6961) -> (30, 131)
  dimension "d3" = 4
  dimension "d4" = 4
  dimension "d5" = 4
  dimension "d6" = 4
  dimension "d7" = 4
  constraint horizontal L1302
  constraint vertical L1303
  constraint horizontal L1304
  constraint vertical L1305
  measures "d3" distance of L3 L1304.end
  measures "d4" horizontal distance of L1.start L1304.end
  measures "d5" vertical distance of L1.end L1302.start
  measures "d6" vertical distance of L0.start L1303.end
  measures "d7" horizontal distance of L0.start L1303.end
sketch "Sketch2" plane through (0, 0, 0) normal (0, 0, 1) x (1, 0, 0)
extrude "Extrude1" add sketch "PV_PWM_heater_v2_4" along normal blind 0.1 contours L0 L1 L2 L3
extrude "Extrude2" add sketch "PV_PWM_heater_v2_4" along normal blind 3 contours L1302 L1303 L1304 L1305
